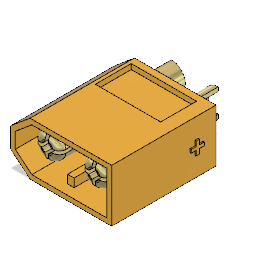
AMASS_XT60-M_1x02_P7.2mm_Vertical (Autodesk Fusion 360 design; units mm, degrees)
Autodesk Fusion 360 part; units mm, degrees
note: some values were not read from the file. Chosen so that the rebuilt part matches the saved one: which bodies a step acts on. Set by a fixed rule: which sketch regions a step uses.
sketch "Sketch19" plane through (0, 0, 0) normal (0, 0, 1) x (1, 0, 0)
  line L0 (0, 0) -> (7.2, 0) construction
  line L1 (7.2, 0) -> (11.35, 0) construction
  line L2 (11.35, -4.05) -> (11.35, 4.05)
  line L3 (11.35, 4.05) -> (-1.15, 4.05)
  line L4 (11.35, -4.05) -> (-1.15, -4.05)
  line L5 (-4.15, 1.55) -> (-4.15, -1.55)
  line L6 (-1.15, 4.05) -> (-4.15, 1.55)
  line L7 (-1.15, -4.05) -> (-4.15, -1.55)
  line L8 (-1.15, 4.05) -> (-4.15, 4.05) construction
  line L9 (-4.15, 4.05) -> (-4.15, 1.55) construction
  line L10 (0, 0) -> (-4.15, 0) construction
  point P0 (3.6, 0)
  dimension "d85" = 7.2
  dimension "d86" = 8.1
  dimension "d87" = 12.5
  dimension "d88" = 12.5
  dimension "d89" = 3.1
  dimension "d90" = 3
  dimension "d91" = 2.5
  dimension "d92" = 3.3
  dimension "d93" = 5
  constraint horizontal L0
  constraint coincident L0.start L10.start
  constraint parallel L0 L1
  constraint vertical L2
  constraint midpoint L1.end L2
  constraint horizontal L3
  constraint horizontal L4
  constraint vertical L5
  constraint perpendicular L5 L8
  constraint perpendicular L8 L9
  constraint midpoint L5 L10.end
  constraint equal L1 L10
  constraint midpoint L0 P0
  measures "d85" distance of L0.start L0.end
  measures "d86" distance of L2.start L2.end
  measures "d87" distance of L2.end L3.end
  measures "d88" distance of L2.start L4.end
  measures "d89" distance of L5.start L5.end
  measures "d90" distance of L3.end L8.end
  measures "d91" distance of L5.start L8.end
extrude "Extrude15" add sketch "Sketch19" along normal blind 16 makes body 1
sketch "Sketch20" plane through (0, 0, 16) normal (0, 0, 1) x (1, 0, 0)
  line L0 (11.35, -4.05) -> (11.35, 4.05)
  line L1 (11.35, 4.05) -> (-1.15, 4.05)
  line L2 (-1.15, 4.05) -> (-4.15, 1.55)
  line L3 (-4.15, 1.55) -> (-4.15, -1.55)
  line L4 (-4.15, -1.55) -> (-1.15, -4.05)
  line L5 (-1.15, -4.05) -> (11.35, -4.05)
  line L6 (-3.4, 1.1987) -> (-3.4, -1.1987)
  line L7 (-3.4, -1.1987) -> (-0.8785, -3.3)
  line L8 (-0.8785, -3.3) -> (10.6, -3.3)
  line L9 (10.6, -3.3) -> (10.6, 3.3)
  line L10 (10.6, 3.3) -> (-0.8785, 3.3)
  line L11 (-0.8785, 3.3) -> (-3.4, 1.1987)
  dimension "d96" = 0.75
extrude "Extrude16" cut sketch "Sketch20" against normal blind 9.3 contours L6 L7 L8 L9 L10 L11 bodies 1
sketch "Sketch21" plane through (0, 0, 6.7) normal (0, 0, 1) x (1, 0, 0)
  line L0 (-0.8785, 3.3) -> (-3.4, 1.1987)
  line L1 (-3.4, 1.1987) -> (-3.4, -1.1987)
  line L2 (-3.4, -1.1987) -> (-0.8785, -3.3)
  line L3 (-0.8785, -3.3) -> (10.6, -3.3)
  line L4 (10.6, -3.3) -> (10.6, 3.3)
  line L5 (10.6, 3.3) -> (-0.8785, 3.3)
  circle A0 centre (7.2, 0) radius 2.15
  circle A1 centre (0, 0) radius 2.15
  point P0 (7.2, 0)
  dimension "d99" = 4.3
  dimension "d100" = 4.3
  constraint coincident P0 A0.centre
  constraint coincident A1.centre origin
  measures "d99" diameter of A0
  measures "d100" diameter of A1
extrude "Extrude17" add sketch "Sketch21" along normal blind 0.35 contours A0 | A1 bodies 1
sketch "Sketch22" plane through (0, 0, 7.05) normal (0, 0, 1) x (1, 0, 0)
  circle A0 centre (7.2, 0) radius 2.15
  circle A1 centre (7.2, 0) radius 1.95
  dimension "d103" = 0.2
sketch "Sketch23" plane through (0, 0, 7.05) normal (0, 0, 1) x (1, 0, 0)
  circle A0 centre (0, 0) radius 2.15
  circle A1 centre (0, 0) radius 1.95
  dimension "d104" = 0.2
extrude "Extrude18" add sketch "Sketch22" sketch "Sketch23" along normal blind 7.55 contours A1 of sketch 2 contours A1 bodies 1
fillet "Fillet1" radius 1 2 edges at (5.382, -0.7052, 14.6) (-1.818, -0.7052, 14.6) on bodies 1
hole "Hole6" at (7.2, 0, 14.6) direction (0, 0, -1) diameter 1.5 depth 7.55 tip angle 118 bodies 1
sketch "Sketch24" plane through (0, 0, 14.6) normal (0, 0, 1) x (1, 0, 0)
  circle A0 centre (7.2, 0) radius 0.75
  circle A1 centre (7.2, 0) radius 0.95
  line L0 (7.45, 2.1472) -> (6.95, 2.1472)
  line L1 (6.95, 2.1472) -> (6.95, -2.1472)
  line L2 (6.95, -2.1472) -> (7.45, -2.1472)
  line L3 (7.45, -2.1472) -> (7.45, 2.1472)
  line L4 (7.45, 2.1472) -> (6.95, -2.1472) construction
  line L5 (6.95, 2.1472) -> (7.45, -2.1472) construction
  line L6 (9.5, -0.25) -> (4.9, -0.25)
  line L7 (4.9, -0.25) -> (4.9, 0.25)
  line L8 (4.9, 0.25) -> (9.5, 0.25)
  line L9 (9.5, 0.25) -> (9.5, -0.25)
  line L10 (9.5, -0.25) -> (4.9, 0.25) construction
  line L11 (4.9, -0.25) -> (9.5, 0.25) construction
  point P0 (7.2, 0)
  point P1 (7.2, 0)
  dimension "d111" = 4.2944
  dimension "d112" = 0.5
  dimension "d113" = 4.6
  dimension "d114" = 0.5
  constraint perpendicular L0 L1
  constraint parallel L0 L2
  constraint parallel L1 L3
  constraint horizontal L0
  constraint coincident L4 P1
  constraint coincident L5 P1
  constraint coincident P0 A0.centre
  constraint perpendicular L6 L7
  constraint parallel L6 L8
  constraint parallel L7 L9
  constraint horizontal L6
  constraint coincident L10 P1
  constraint coincident L11 P1
  constraint coincident P1 P0
  measures "d111" distance of L0.end L1.end
  measures "d112" distance of L1.end L2.end
  measures "d113" distance of L7.end L8.end
  measures "d114" distance of L6.end L7.end
extrude "Extrude19" cut sketch "Sketch24" against normal blind 7.55 contours A0 L3 L6 L8 | A0 A1 L6 L8 | A0 L1 L3 L8 | A0 A1 L1 L3 | L1 L3 L6 L8 | A1 L6 L8 L9 | A0 A1 L1 L3 | A0 L1 L3 L6 | A1 L0 L1 L3 | A0 L1 L6 L8 | A1 L1 L2 L3 | A0 A1 L6 L8 | A1 L6 L7 L8 bodies 1
hole "Hole7" at (0, 0, 14.6) direction (0, 0, -1) diameter 1.5 depth 7.55 tip angle 118 bodies 1
sketch "Sketch25" plane through (0, 0, 14.6) normal (0, 0, 1) x (1, 0, 0)
  circle A0 centre (0, 0) radius 0.75
  circle A1 centre (0, 0) radius 0.95
  line L0 (0.25, 2.1275) -> (-0.25, 2.1275)
  line L1 (-0.25, 2.1275) -> (-0.25, -2.1275)
  line L2 (-0.25, -2.1275) -> (0.25, -2.1275)
  line L3 (0.25, -2.1275) -> (0.25, 2.1275)
  line L4 (0.25, 2.1275) -> (-0.25, -2.1275) construction
  line L5 (-0.25, 2.1275) -> (0.25, -2.1275) construction
  line L6 (2.1235, 0.25) -> (-2.1235, 0.25)
  line L7 (-2.1235, 0.25) -> (-2.1235, -0.25)
  line L8 (-2.1235, -0.25) -> (2.1235, -0.25)
  line L9 (2.1235, -0.25) -> (2.1235, 0.25)
  line L10 (2.1235, 0.25) -> (-2.1235, -0.25) construction
  line L11 (-2.1235, 0.25) -> (2.1235, -0.25) construction
  dimension "d120" = 0.5
  dimension "d121" = 4.2551
  dimension "d122" = 4.247
  dimension "d123" = 0.5
  constraint perpendicular L0 L1
  constraint parallel L0 L2
  constraint parallel L1 L3
  constraint horizontal L0
  constraint coincident L4 A0.centre
  constraint coincident L5 A0.centre
  constraint coincident A0.centre A1.centre
  constraint perpendicular L6 L7
  constraint parallel L6 L8
  constraint parallel L7 L9
  constraint horizontal L6
  constraint coincident L10 A0.centre
  constraint coincident L11 A0.centre
  measures "d120" distance of L1.end L2.end
  measures "d121" distance of L0.end L1.end
  measures "d122" distance of L7.end L8.end
  measures "d123" distance of L6.end L7.end
extrude "Extrude20" cut sketch "Sketch25" against normal blind 7.55 contours A0 L3 L6 L8 | A0 A1 L6 L8 | A0 L1 L3 L6 | A0 A1 L1 L3 | A1 L6 L8 L9 | L1 L3 L6 L8 | A0 A1 L1 L3 | A0 L1 L3 L8 | A1 L0 L1 L3 | A0 L1 L6 L8 | A1 L1 L2 L3 | A0 A1 L6 L8 | A1 L6 L7 L8 bodies 1
sketch "Sketch26" plane through (0, 0, 6.7) normal (0, 0, 1) x (1, 0, 0)
  circle A0 centre (7.2, 0) radius 2.15
  circle A1 centre (0, 0) radius 2.15
  line L0 (-0.8785, 3.3) -> (-3.4, 1.1987)
  line L1 (-3.4, 1.1987) -> (-3.4, -1.1987)
  line L2 (-3.4, -1.1987) -> (-0.8785, -3.3)
  line L3 (-0.8785, -3.3) -> (10.6, -3.3)
  line L4 (10.6, -3.3) -> (10.6, 3.3)
  line L5 (10.6, 3.3) -> (-0.8785, 3.3)
  line L6 (4.25, 2) -> (2.95, 2)
  line L7 (2.95, 2) -> (2.95, -2)
  line L8 (2.95, -2) -> (4.25, -2)
  line L9 (4.25, -2) -> (4.25, 2)
  line L10 (4.25, 2) -> (2.95, -2) construction
  line L11 (2.95, 2) -> (4.25, -2) construction
  point P0 (3.6, 0)
  point P1 (3.6, 0)
  dimension "d126" = 1.3
  dimension "d127" = 4
  constraint perpendicular L6 L7
  constraint parallel L6 L8
  constraint parallel L7 L9
  constraint horizontal L6
  constraint coincident L10 P1
  constraint coincident L11 P1
  constraint coincident P1 P0
  measures "d126" distance of L7.end L8.end
  measures "d127" distance of L6.end L7.end
extrude "Extrude21" cut sketch "Sketch26" against normal blind 1 contours L6 L7 L8 L9 bodies 1
sketch "Sketch27" plane through (0, 0, 6.7) normal (0, 0, 1) x (1, 0, 0)
  line L0 (2.95, 2) -> (4.25, 2)
  line L1 (4.25, 2) -> (4.25, -2)
  line L2 (4.25, -2) -> (2.95, -2)
  line L3 (2.95, -2) -> (2.95, 2)
  circle A0 centre (7.2, 0) radius 2.15
  circle A1 centre (0, 0) radius 2.15
  line L4 (-0.8785, 3.3) -> (-3.4, 1.1987)
  line L5 (-3.4, 1.1987) -> (-3.4, -1.1987)
  line L6 (-3.4, -1.1987) -> (-0.8785, -3.3)
  line L7 (-0.8785, -3.3) -> (10.6, -3.3)
  line L8 (10.6, -3.3) -> (10.6, 3.3)
  line L9 (10.6, 3.3) -> (-0.8785, 3.3)
  line L10 (3.6, -2) -> (3.6, -3.3) construction
  line L11 (4.1, -2) -> (3.1, -2)
  line L12 (3.1, -2) -> (3.1, -3.3)
  line L13 (3.1, -3.3) -> (4.1, -3.3)
  line L14 (4.1, -3.3) -> (4.1, -2)
  line L15 (4.1, -2) -> (3.1, -3.3) construction
  line L16 (3.1, -2) -> (4.1, -3.3) construction
  point P0 (3.6, -2)
  point P1 (3.6, -2.65)
  dimension "d130" = 1
  dimension "d131" = 1.3
  constraint midpoint L2 P0
  constraint coincident P0 L10.start
  constraint coincident L7 L10.end
  constraint perpendicular L11 L12
  constraint parallel L11 L13
  constraint parallel L12 L14
  constraint horizontal L11
  constraint coincident L15 P1
  constraint coincident L16 P1
  constraint midpoint L10 P1
  measures "d130" distance of L12.end L13.end
  measures "d131" distance of L11.end L12.end
extrude "Extrude22" add sketch "Sketch27" along normal blind 7.8 contours L2 L7 L11 L12 L13 L14 bodies 1
sketch "Sketch28" plane through (0, 0, 0) normal (0, 0, 1) x (1, 0, 0)
  circle A0 centre (0, 0) radius 3
  circle A1 centre (7.2, 0) radius 3
  point P0 (7.2, 0)
  dimension "d134" = 6
  dimension "d135" = 6
  constraint coincident A0.centre origin
  constraint coincident P0 A1.centre
  measures "d134" diameter of A0
  measures "d135" diameter of A1
extrude "Extrude23" cut sketch "Sketch28" along normal blind 3 bodies 1
sketch "Sketch29" plane through (0, 0, 3) normal (0, 0, -1) x (-1, 0, 0)
  circle A0 centre (-7.2, 0) radius 3
  circle A1 centre (-7.2, 0) radius 2.15
  circle A2 centre (0, 0) radius 2.15
  dimension "d138" = 4.3
  dimension "d139" = 4.3
  constraint concentric A0 A1
  constraint coincident A2.centre origin
  measures "d138" diameter of A1
  measures "d139" diameter of A2
extrude "Extrude24" add sketch "Sketch29" along normal blind 7.5 contours A1 | A2 bodies 1
hole "Hole8" at (7.2, 0, -4.5) direction (0, 0, 1) diameter 3 depth 6 tip angle 118 bodies 1
hole "Hole9" at (0, 0, -4.5) direction (0, 0, 1) diameter 3 depth 6 tip angle 118 bodies 1
ref_plane "WorkPlane3" through (0, -2.15, -0.75) normal (0, -1, 0) x (-1, 0, 0)
sketch "Sketch30" plane through (0, -2.15, -0.75) normal (0, -1, 0) x (1, 0, 0)
  line L0 (0, -3.75) -> (-2.9, -3.75)
  line L1 (-2.9, -3.75) -> (-2.9, -0.75)
  line L2 (-2.9, -0.75) -> (0, -0.75)
  line L3 (0, -0.75) -> (0, -3.75)
  line L4 (1.5, -3.75) -> (-1.5, -3.75)
  dimension "d149" = 3
  dimension "d150" = 2.9
  constraint horizontal L0
  constraint vertical L1
  constraint horizontal L2
  constraint vertical L3
  constraint midpoint L0.start L4
  measures "d149" distance of L0.start L2.end
  measures "d150" distance of L0.start L0.end
extrude "Extrude25" cut sketch "Sketch30" against normal blind 5.1 bodies 1
sketch "Sketch31" plane through (0, -2.15, -0.75) normal (0, -1, 0) x (1, 0, 0)
  line L0 (7.2, -3.75) -> (10.5241, -3.75)
  line L1 (10.5241, -3.75) -> (10.5241, -0.75)
  line L2 (10.5241, -0.75) -> (7.2, -0.75)
  line L3 (7.2, -0.75) -> (7.2, -3.75)
  line L4 (8.7, -3.75) -> (5.7, -3.75)
  dimension "d153" = 3.3241
  dimension "d154" = 3
  constraint horizontal L0
  constraint vertical L1
  constraint horizontal L2
  constraint vertical L3
  constraint midpoint L0.start L4
  measures "d153" distance of L0.start L0.end
  measures "d154" distance of L0.start L2.end
extrude "Extrude26" cut sketch "Sketch31" against normal blind 5.5 bodies 1
sketch "Sketch32" plane through (11.35, 0, 0) normal (1, 0, 0) x (0, 0, -1)
  line L0 (0, -4.05) -> (0, 4.05)
  line L1 (0, 4.05) -> (-16, 4.05)
  line L2 (-16, 4.05) -> (-16, -4.05)
  line L3 (-16, -4.05) -> (0, -4.05)
  line L4 (0, 0) -> (-2, 0) construction
  line L5 (0, 1.55) -> (-16, 1.55)
  line L6 (-2, -0.25) -> (-2, 0.25)
  line L7 (-2, 0.25) -> (-2.75, 0.25)
  line L8 (-2.75, 0.25) -> (-2.75, 1)
  line L9 (-2.75, 1) -> (-3.25, 1)
  line L10 (-3.25, 1) -> (-3.25, 0.25)
  line L11 (-3.25, 0.25) -> (-4, 0.25)
  line L12 (-4, 0.25) -> (-4, -0.25)
  line L13 (-4, -0.25) -> (-3.25, -0.25)
  line L14 (-3.25, -0.25) -> (-3.25, -1)
  line L15 (-3.25, -1) -> (-2.75, -1)
  line L16 (-2.75, -1) -> (-2.75, -0.25)
  line L17 (-2.75, -0.25) -> (-2, -0.25)
  dimension "d157" = 2
  dimension "d158" = 0.5
  dimension "d159" = 0.75
  constraint horizontal L4
  constraint coincident L4.start origin
  constraint perpendicular L5 L6
  constraint perpendicular L5 L8
  constraint perpendicular L8 L9
  constraint perpendicular L9 L10
  constraint perpendicular L10 L11
  constraint perpendicular L9 L12
  constraint perpendicular L10 L13
  constraint perpendicular L9 L14
  constraint perpendicular L10 L15
  constraint perpendicular L15 L16
  constraint perpendicular L6 L17
  constraint equal L12 L15
  constraint equal L6 L15
  constraint equal L6 L9
  constraint equal L16 L17
  constraint equal L7 L17
  constraint equal L7 L8
  constraint equal L8 L10
  constraint equal L10 L11
  constraint equal L11 L13
  constraint equal L13 L14
  constraint midpoint L4.end L6
  measures "d157" distance of L4.start L4.end
  measures "d158" distance of L8.end L9.end
  measures "d159" distance of L9.end L10.end
extrude "Extrude27" add sketch "Sketch32" along normal blind 0.2 contours L6 L7 L8 L9 L10 L11 L12 L13 L14 L15 L16 L17 bodies 1
sketch "Sketch33" plane through (-4.15, 0, 0) normal (-1, 0, 0) x (0, 0, 1)
  line L0 (0, 1.55) -> (0, -1.55)
  line L1 (0, -1.55) -> (16, -1.55)
  line L2 (16, -1.55) -> (16, 1.55)
  line L3 (16, 1.55) -> (0, 1.55)
  line L4 (0, 0) -> (3, 0) construction
  line L5 (3, 1) -> (3.2, 1)
  line L6 (3.2, 1) -> (3.2, -1)
  line L7 (3.2, -1) -> (3, -1)
  line L8 (3, -1) -> (3, 1)
  dimension "d162" = 3
  dimension "d165" = 0.2
  dimension "d166" = 2
  constraint coincident L4.start origin
  constraint perpendicular L0 L4
  constraint horizontal L5
  constraint vertical L6
  constraint horizontal L7
  constraint vertical L8
  constraint midpoint L4.end L8
  measures "d162" distance of L4.start L4.end
  measures "d165" distance of L6.end L7.end
  measures "d166" distance of L5.end L6.end
extrude "Extrude28" add sketch "Sketch33" along normal blind 0.2 contours L5 L6 L7 L8 bodies 1
sketch "Sketch34" plane through (0, 4.05, 0) normal (0, 1, 0) x (-1, 0, 0)
  line L0 (-11.35, 0) -> (1.15, 0)
  line L1 (1.15, 0) -> (1.15, 16)
  line L2 (1.15, 16) -> (-11.35, 16)
  line L3 (-11.35, 16) -> (-11.35, 0)
  line L4 (-11.35, 1) -> (-9.35, 1) construction
  line L5 (-9.35, 1) -> (-9.35, 0) construction
  line L6 (-9.35, 1) -> (0.65, 1)
  line L7 (0.65, 1) -> (0.65, 6.5)
  line L8 (0.65, 6.5) -> (-9.35, 6.5)
  line L9 (-9.35, 6.5) -> (-9.35, 1)
  dimension "d169" = 1
  dimension "d170" = 2
  dimension "d171" = 10
  dimension "d172" = 5.5
  constraint coincident L3 L4.start
  constraint perpendicular L3 L4
  constraint coincident L0 L5.end
  constraint horizontal L6
  constraint vertical L7
  constraint horizontal L8
  constraint vertical L9
  measures "d169" distance of L4.end L5.end
  measures "d170" distance of L4.start L4.end
  measures "d171" distance of L4.end L6.end
  measures "d172" distance of L4.end L8.end
extrude "Extrude29" cut sketch "Sketch34" against normal blind 0.8 contours L6 L7 L8 L9 bodies 1
sketch "Sketch35" plane through (0, -4.05, 0) normal (0, -1, 0) x (1, 0, 0)
  line L0 (-1.15, 0) -> (11.35, 0)
  line L1 (11.35, 0) -> (11.35, 16)
  line L2 (11.35, 16) -> (-1.15, 16)
  line L3 (-1.15, 16) -> (-1.15, 0)
  line L4 (11.35, 1) -> (9.35, 1) construction
  line L5 (9.35, 1) -> (9.35, 0) construction
  line L6 (9.651, 1) -> (-0.349, 1)
  line L7 (-0.349, 1) -> (-0.349, 6.5)
  line L8 (-0.349, 6.5) -> (9.651, 6.5)
  line L9 (9.651, 6.5) -> (9.651, 1)
  dimension "d175" = 2
  dimension "d176" = 1
  dimension "d177" = 10
  dimension "d178" = 5.5
  constraint coincident L1 L4.start
  constraint perpendicular L1 L4
  constraint coincident L0 L5.end
  constraint perpendicular L0 L5
  constraint horizontal L6
  constraint vertical L7
  constraint horizontal L8
  constraint vertical L9
  constraint coincident L4 L6.start
  measures "d175" distance of L4.start L4.end
  measures "d176" distance of L4.end L5.end
  measures "d177" distance of L6.start L6.end
  measures "d178" distance of L6.start L8.end
extrude "Extrude30" cut sketch "Sketch35" against normal blind 0.8 contours L6 L7 L8 L9 bodies 1
split "Split3" by face at (6.9375, 2.1339, -1) of body 1 bodies 1 makes body 2 at (6.617, -4.05, 12.8333)
split "Split4" by face at (0.2673, -2.1333, -1) of body 2 bodies 2 makes body 3 at (6.617, -4.05, 12.8333)
named bodies: "Pin2", "Pin1"
